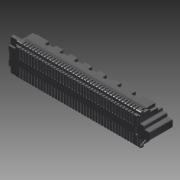
# Autodesk Inventor part: SS4-40_socket
Saved by Autodesk Inventor 2016 (Build 200138000, 138)
## iProperties
Category: PARTsolutions
Company: SAMTEC
Created: 2016-06-07
Part Number: SS4-40_socket
Catalog Web Link: www.cadenas.de
Description: SS4--Socket
Vendor: SAMTEC
Document SubType Name: Modeling
Designer: psAdmin
Manufacturer: SAMTEC
Mass: 0.109161 g
Surface Area: 7.02926 cm^2
Volume: 0.109161 cm^3
Density: 1 g/cm^3
Material: Generic
Appearance: PSOLRGB-175-175-175
PSOL_IDENT_0: {$CADENAS_DATA\23d-libs\samtec\modelling\ss4\parts\ss4_socket.prj},174 {VTYP=3D},{NB=SS4-40_socket},
PSOL_IDENT_1: {LINA=SS4-40_socket},{NN=SS4-},{DATE=07.12.2015 15:39:44},{GEOMDATE=07.12.2015 15:39:00},{VERSION=},
PSOL_IDENT_2: {LINEID=10},{LINESUBID=-1},{WBVAR=POS,LOPT}  {NB=SS4-40_socket},{LINA=SS4-40_socket},{KT=DUMMY},{PN=
PSOL_IDENT_3: SS4-40},{SERIES=SS4},{POSALG=   '10' , '-10' , '15' , '-15' , '20' , '-20' , '30' , '-30' , '40' , '
PSOL_IDENT_4: -40' ,  '50' , '-50'   },{POS=40},{ROPT=D},{LOPT=},{A=17.460},{BH=0.500},{K=2.725},{L=19.540},{W=4.3
PSOL_IDENT_5: 50},{HOLE=0.585},{PINS=40},{PINW=0.166},{PITCH=0.40},{LOPTPN=}
NN: SS4-
NT: Socket
NB: SS4-40_socket
NBSYN: $PN._socket
LINA: SS4-40_socket
PN: SS4-40
SERIES: SS4
POS: -40
ROPT: D
LOPT: Not Selected
A: 17.460
BH: 0.500
K: 2.725
L: 19.540
W: 4.350
HOLE: 0.585
PINW: 0.166
PITCH: 0.40
SUPPLIER: SAMTEC
ARTICLENO: SS4-40_socket
BOMINFO: SS4-40_socket
CREATOR: CADENAS GmbH
Title: SS4-40_socket
Author: Cadenas PARTsolutions
Comments: Socket
Autodesk Inventor part; units mm, degrees
sketch "Sketch_1" plane through (0, 0, 0) normal (0, 1, 0) x (1, 0, 0)
  line L0 (-9.56, -0.5) -> (-9.56, -2.175)
  line L1 (-9.56, -2.175) -> (8.58, -2.175)
  line L2 (8.58, -2.175) -> (8.58, -0.5)
  line L3 (8.58, -0.5) -> (8.18, -0.5)
  line L4 (8.18, -0.5) -> (8.18, 0.5)
  line L5 (8.18, 0.5) -> (8.58, 0.5)
  line L6 (8.58, 0.5) -> (8.58, 2.175)
  line L7 (8.58, 2.175) -> (-9.56, 2.175)
  line L8 (-9.56, 2.175) -> (-9.56, 0.5)
  line L9 (-9.56, 0.5) -> (-9.46, 0.5)
  line L10 (-9.46, 0.5) -> (-9.46, -0.5)
  line L11 (-9.46, -0.5) -> (-9.56, -0.5)
  line L12 (7.717, -0.705) -> (7.717, -1.29)
  line L13 (7.717, -1.29) -> (7.883, -1.29)
  line L14 (7.883, -1.29) -> (7.883, -0.705)
  line L15 (7.883, -0.705) -> (7.717, -0.705)
  line L16 (7.717, 1.29) -> (7.717, 0.705)
  line L17 (7.717, 0.705) -> (7.883, 0.705)
  line L18 (7.883, 0.705) -> (7.883, 1.29)
  line L19 (7.883, 1.29) -> (7.717, 1.29)
  line L20 (7.317, -0.705) -> (7.317, -1.29)
  line L21 (7.317, -1.29) -> (7.483, -1.29)
  line L22 (7.483, -1.29) -> (7.483, -0.705)
  line L23 (7.483, -0.705) -> (7.317, -0.705)
  line L24 (7.317, 1.29) -> (7.317, 0.705)
  line L25 (7.317, 0.705) -> (7.483, 0.705)
  line L26 (7.483, 0.705) -> (7.483, 1.29)
  line L27 (7.483, 1.29) -> (7.317, 1.29)
  line L28 (6.917, -0.705) -> (6.917, -1.29)
  line L29 (6.917, -1.29) -> (7.083, -1.29)
  line L30 (7.083, -1.29) -> (7.083, -0.705)
  line L31 (7.083, -0.705) -> (6.917, -0.705)
  line L32 (6.917, 1.29) -> (6.917, 0.705)
  line L33 (6.917, 0.705) -> (7.083, 0.705)
  line L34 (7.083, 0.705) -> (7.083, 1.29)
  line L35 (7.083, 1.29) -> (6.917, 1.29)
  line L36 (6.517, -0.705) -> (6.517, -1.29)
  line L37 (6.517, -1.29) -> (6.683, -1.29)
  line L38 (6.683, -1.29) -> (6.683, -0.705)
  line L39 (6.683, -0.705) -> (6.517, -0.705)
  line L40 (6.517, 1.29) -> (6.517, 0.705)
  line L41 (6.517, 0.705) -> (6.683, 0.705)
  line L42 (6.683, 0.705) -> (6.683, 1.29)
  line L43 (6.683, 1.29) -> (6.517, 1.29)
  line L44 (6.117, -0.705) -> (6.117, -1.29)
  line L45 (6.117, -1.29) -> (6.283, -1.29)
  line L46 (6.283, -1.29) -> (6.283, -0.705)
  line L47 (6.283, -0.705) -> (6.117, -0.705)
  line L48 (6.117, 1.29) -> (6.117, 0.705)
  line L49 (6.117, 0.705) -> (6.283, 0.705)
  line L50 (6.283, 0.705) -> (6.283, 1.29)
  line L51 (6.283, 1.29) -> (6.117, 1.29)
  line L52 (5.717, -0.705) -> (5.717, -1.29)
  line L53 (5.717, -1.29) -> (5.883, -1.29)
  line L54 (5.883, -1.29) -> (5.883, -0.705)
  line L55 (5.883, -0.705) -> (5.717, -0.705)
  line L56 (5.717, 1.29) -> (5.717, 0.705)
  line L57 (5.717, 0.705) -> (5.883, 0.705)
  line L58 (5.883, 0.705) -> (5.883, 1.29)
  line L59 (5.883, 1.29) -> (5.717, 1.29)
  line L60 (5.317, -0.705) -> (5.317, -1.29)
  line L61 (5.317, -1.29) -> (5.483, -1.29)
  line L62 (5.483, -1.29) -> (5.483, -0.705)
  line L63 (5.483, -0.705) -> (5.317, -0.705)
  line L64 (5.317, 1.29) -> (5.317, 0.705)
  line L65 (5.317, 0.705) -> (5.483, 0.705)
  line L66 (5.483, 0.705) -> (5.483, 1.29)
  line L67 (5.483, 1.29) -> (5.317, 1.29)
  line L68 (4.917, -0.705) -> (4.917, -1.29)
  line L69 (4.917, -1.29) -> (5.083, -1.29)
  line L70 (5.083, -1.29) -> (5.083, -0.705)
  line L71 (5.083, -0.705) -> (4.917, -0.705)
  line L72 (4.917, 1.29) -> (4.917, 0.705)
  line L73 (4.917, 0.705) -> (5.083, 0.705)
  line L74 (5.083, 0.705) -> (5.083, 1.29)
  line L75 (5.083, 1.29) -> (4.917, 1.29)
  line L76 (4.517, -0.705) -> (4.517, -1.29)
  line L77 (4.517, -1.29) -> (4.683, -1.29)
  line L78 (4.683, -1.29) -> (4.683, -0.705)
  line L79 (4.683, -0.705) -> (4.517, -0.705)
  line L80 (4.517, 1.29) -> (4.517, 0.705)
  line L81 (4.517, 0.705) -> (4.683, 0.705)
  line L82 (4.683, 0.705) -> (4.683, 1.29)
  line L83 (4.683, 1.29) -> (4.517, 1.29)
  line L84 (4.117, -0.705) -> (4.117, -1.29)
  line L85 (4.117, -1.29) -> (4.283, -1.29)
  line L86 (4.283, -1.29) -> (4.283, -0.705)
  line L87 (4.283, -0.705) -> (4.117, -0.705)
  line L88 (4.117, 1.29) -> (4.117, 0.705)
  line L89 (4.117, 0.705) -> (4.283, 0.705)
  line L90 (4.283, 0.705) -> (4.283, 1.29)
  line L91 (4.283, 1.29) -> (4.117, 1.29)
  line L92 (3.717, -0.705) -> (3.717, -1.29)
  line L93 (3.717, -1.29) -> (3.883, -1.29)
  line L94 (3.883, -1.29) -> (3.883, -0.705)
  line L95 (3.883, -0.705) -> (3.717, -0.705)
  line L96 (3.717, 1.29) -> (3.717, 0.705)
  line L97 (3.717, 0.705) -> (3.883, 0.705)
  line L98 (3.883, 0.705) -> (3.883, 1.29)
  line L99 (3.883, 1.29) -> (3.717, 1.29)
  line L100 (3.317, -0.705) -> (3.317, -1.29)
  line L101 (3.317, -1.29) -> (3.483, -1.29)
  line L102 (3.483, -1.29) -> (3.483, -0.705)
  line L103 (3.483, -0.705) -> (3.317, -0.705)
  line L104 (3.317, 1.29) -> (3.317, 0.705)
  line L105 (3.317, 0.705) -> (3.483, 0.705)
  line L106 (3.483, 0.705) -> (3.483, 1.29)
  line L107 (3.483, 1.29) -> (3.317, 1.29)
  line L108 (2.917, -0.705) -> (2.917, -1.29)
  line L109 (2.917, -1.29) -> (3.083, -1.29)
  line L110 (3.083, -1.29) -> (3.083, -0.705)
  line L111 (3.083, -0.705) -> (2.917, -0.705)
  line L112 (2.917, 1.29) -> (2.917, 0.705)
  line L113 (2.917, 0.705) -> (3.083, 0.705)
  line L114 (3.083, 0.705) -> (3.083, 1.29)
  line L115 (3.083, 1.29) -> (2.917, 1.29)
  line L116 (2.517, -0.705) -> (2.517, -1.29)
  line L117 (2.517, -1.29) -> (2.683, -1.29)
  line L118 (2.683, -1.29) -> (2.683, -0.705)
  line L119 (2.683, -0.705) -> (2.517, -0.705)
  line L120 (2.517, 1.29) -> (2.517, 0.705)
  line L121 (2.517, 0.705) -> (2.683, 0.705)
  line L122 (2.683, 0.705) -> (2.683, 1.29)
  line L123 (2.683, 1.29) -> (2.517, 1.29)
  line L124 (2.117, -0.705) -> (2.117, -1.29)
  line L125 (2.117, -1.29) -> (2.283, -1.29)
  line L126 (2.283, -1.29) -> (2.283, -0.705)
  line L127 (2.283, -0.705) -> (2.117, -0.705)
  line L128 (2.117, 1.29) -> (2.117, 0.705)
  line L129 (2.117, 0.705) -> (2.283, 0.705)
  line L130 (2.283, 0.705) -> (2.283, 1.29)
  line L131 (2.283, 1.29) -> (2.117, 1.29)
  line L132 (1.717, -0.705) -> (1.717, -1.29)
  line L133 (1.717, -1.29) -> (1.883, -1.29)
  line L134 (1.883, -1.29) -> (1.883, -0.705)
  line L135 (1.883, -0.705) -> (1.717, -0.705)
  line L136 (1.717, 1.29) -> (1.717, 0.705)
  line L137 (1.717, 0.705) -> (1.883, 0.705)
  line L138 (1.883, 0.705) -> (1.883, 1.29)
  line L139 (1.883, 1.29) -> (1.717, 1.29)
  line L140 (1.317, -0.705) -> (1.317, -1.29)
  line L141 (1.317, -1.29) -> (1.483, -1.29)
  line L142 (1.483, -1.29) -> (1.483, -0.705)
  line L143 (1.483, -0.705) -> (1.317, -0.705)
  line L144 (1.317, 1.29) -> (1.317, 0.705)
  line L145 (1.317, 0.705) -> (1.483, 0.705)
  line L146 (1.483, 0.705) -> (1.483, 1.29)
  line L147 (1.483, 1.29) -> (1.317, 1.29)
  line L148 (0.917, -0.705) -> (0.917, -1.29)
  line L149 (0.917, -1.29) -> (1.083, -1.29)
  line L150 (1.083, -1.29) -> (1.083, -0.705)
  line L151 (1.083, -0.705) -> (0.917, -0.705)
  line L152 (0.917, 1.29) -> (0.917, 0.705)
  line L153 (0.917, 0.705) -> (1.083, 0.705)
  line L154 (1.083, 0.705) -> (1.083, 1.29)
  line L155 (1.083, 1.29) -> (0.917, 1.29)
  line L156 (0.517, -0.705) -> (0.517, -1.29)
  line L157 (0.517, -1.29) -> (0.683, -1.29)
  line L158 (0.683, -1.29) -> (0.683, -0.705)
  line L159 (0.683, -0.705) -> (0.517, -0.705)
  line L160 (0.517, 1.29) -> (0.517, 0.705)
  line L161 (0.517, 0.705) -> (0.683, 0.705)
  line L162 (0.683, 0.705) -> (0.683, 1.29)
  line L163 (0.683, 1.29) -> (0.517, 1.29)
  line L164 (0.117, -0.705) -> (0.117, -1.29)
  line L165 (0.117, -1.29) -> (0.283, -1.29)
  line L166 (0.283, -1.29) -> (0.283, -0.705)
  line L167 (0.283, -0.705) -> (0.117, -0.705)
  line L168 (0.117, 1.29) -> (0.117, 0.705)
  line L169 (0.117, 0.705) -> (0.283, 0.705)
  line L170 (0.283, 0.705) -> (0.283, 1.29)
  line L171 (0.283, 1.29) -> (0.117, 1.29)
  line L172 (-0.283, -0.705) -> (-0.283, -1.29)
  line L173 (-0.283, -1.29) -> (-0.117, -1.29)
  line L174 (-0.117, -1.29) -> (-0.117, -0.705)
  line L175 (-0.117, -0.705) -> (-0.283, -0.705)
  line L176 (-0.283, 1.29) -> (-0.283, 0.705)
  line L177 (-0.283, 0.705) -> (-0.117, 0.705)
  line L178 (-0.117, 0.705) -> (-0.117, 1.29)
  line L179 (-0.117, 1.29) -> (-0.283, 1.29)
  line L180 (-0.683, -0.705) -> (-0.683, -1.29)
  line L181 (-0.683, -1.29) -> (-0.517, -1.29)
  line L182 (-0.517, -1.29) -> (-0.517, -0.705)
  line L183 (-0.517, -0.705) -> (-0.683, -0.705)
  line L184 (-0.683, 1.29) -> (-0.683, 0.705)
  line L185 (-0.683, 0.705) -> (-0.517, 0.705)
  line L186 (-0.517, 0.705) -> (-0.517, 1.29)
  line L187 (-0.517, 1.29) -> (-0.683, 1.29)
  line L188 (-1.083, -0.705) -> (-1.083, -1.29)
  line L189 (-1.083, -1.29) -> (-0.917, -1.29)
  line L190 (-0.917, -1.29) -> (-0.917, -0.705)
  line L191 (-0.917, -0.705) -> (-1.083, -0.705)
  line L192 (-1.083, 1.29) -> (-1.083, 0.705)
  line L193 (-1.083, 0.705) -> (-0.917, 0.705)
  line L194 (-0.917, 0.705) -> (-0.917, 1.29)
  line L195 (-0.917, 1.29) -> (-1.083, 1.29)
  line L196 (-1.483, -0.705) -> (-1.483, -1.29)
  line L197 (-1.483, -1.29) -> (-1.317, -1.29)
  line L198 (-1.317, -1.29) -> (-1.317, -0.705)
  line L199 (-1.317, -0.705) -> (-1.483, -0.705)
  line L200 (-1.483, 1.29) -> (-1.483, 0.705)
  line L201 (-1.483, 0.705) -> (-1.317, 0.705)
  line L202 (-1.317, 0.705) -> (-1.317, 1.29)
  line L203 (-1.317, 1.29) -> (-1.483, 1.29)
  line L204 (-1.883, -0.705) -> (-1.883, -1.29)
  line L205 (-1.883, -1.29) -> (-1.717, -1.29)
  line L206 (-1.717, -1.29) -> (-1.717, -0.705)
  line L207 (-1.717, -0.705) -> (-1.883, -0.705)
  line L208 (-1.883, 1.29) -> (-1.883, 0.705)
  line L209 (-1.883, 0.705) -> (-1.717, 0.705)
  line L210 (-1.717, 0.705) -> (-1.717, 1.29)
  line L211 (-1.717, 1.29) -> (-1.883, 1.29)
  line L212 (-2.283, -0.705) -> (-2.283, -1.29)
  line L213 (-2.283, -1.29) -> (-2.117, -1.29)
  line L214 (-2.117, -1.29) -> (-2.117, -0.705)
  line L215 (-2.117, -0.705) -> (-2.283, -0.705)
  line L216 (-2.283, 1.29) -> (-2.283, 0.705)
  line L217 (-2.283, 0.705) -> (-2.117, 0.705)
  line L218 (-2.117, 0.705) -> (-2.117, 1.29)
  line L219 (-2.117, 1.29) -> (-2.283, 1.29)
  line L220 (-2.683, -0.705) -> (-2.683, -1.29)
  line L221 (-2.683, -1.29) -> (-2.517, -1.29)
  line L222 (-2.517, -1.29) -> (-2.517, -0.705)
  line L223 (-2.517, -0.705) -> (-2.683, -0.705)
  line L224 (-2.683, 1.29) -> (-2.683, 0.705)
  line L225 (-2.683, 0.705) -> (-2.517, 0.705)
  line L226 (-2.517, 0.705) -> (-2.517, 1.29)
  line L227 (-2.517, 1.29) -> (-2.683, 1.29)
  line L228 (-3.083, -0.705) -> (-3.083, -1.29)
  line L229 (-3.083, -1.29) -> (-2.917, -1.29)
  line L230 (-2.917, -1.29) -> (-2.917, -0.705)
  line L231 (-2.917, -0.705) -> (-3.083, -0.705)
  line L232 (-3.083, 1.29) -> (-3.083, 0.705)
  line L233 (-3.083, 0.705) -> (-2.917, 0.705)
  line L234 (-2.917, 0.705) -> (-2.917, 1.29)
  line L235 (-2.917, 1.29) -> (-3.083, 1.29)
  line L236 (-3.483, -0.705) -> (-3.483, -1.29)
  line L237 (-3.483, -1.29) -> (-3.317, -1.29)
  line L238 (-3.317, -1.29) -> (-3.317, -0.705)
  line L239 (-3.317, -0.705) -> (-3.483, -0.705)
  line L240 (-3.483, 1.29) -> (-3.483, 0.705)
  line L241 (-3.483, 0.705) -> (-3.317, 0.705)
  line L242 (-3.317, 0.705) -> (-3.317, 1.29)
  line L243 (-3.317, 1.29) -> (-3.483, 1.29)
  line L244 (-3.883, -0.705) -> (-3.883, -1.29)
  line L245 (-3.883, -1.29) -> (-3.717, -1.29)
  line L246 (-3.717, -1.29) -> (-3.717, -0.705)
  line L247 (-3.717, -0.705) -> (-3.883, -0.705)
  line L248 (-3.883, 1.29) -> (-3.883, 0.705)
  line L249 (-3.883, 0.705) -> (-3.717, 0.705)
  line L250 (-3.717, 0.705) -> (-3.717, 1.29)
  line L251 (-3.717, 1.29) -> (-3.883, 1.29)
  line L252 (-4.283, -0.705) -> (-4.283, -1.29)
  line L253 (-4.283, -1.29) -> (-4.117, -1.29)
  line L254 (-4.117, -1.29) -> (-4.117, -0.705)
  line L255 (-4.117, -0.705) -> (-4.283, -0.705)
  line L256 (-4.283, 1.29) -> (-4.283, 0.705)
  line L257 (-4.283, 0.705) -> (-4.117, 0.705)
  line L258 (-4.117, 0.705) -> (-4.117, 1.29)
  line L259 (-4.117, 1.29) -> (-4.283, 1.29)
  line L260 (-4.683, -0.705) -> (-4.683, -1.29)
  line L261 (-4.683, -1.29) -> (-4.517, -1.29)
  line L262 (-4.517, -1.29) -> (-4.517, -0.705)
  line L263 (-4.517, -0.705) -> (-4.683, -0.705)
  line L264 (-4.683, 1.29) -> (-4.683, 0.705)
  line L265 (-4.683, 0.705) -> (-4.517, 0.705)
  line L266 (-4.517, 0.705) -> (-4.517, 1.29)
  line L267 (-4.517, 1.29) -> (-4.683, 1.29)
  line L268 (-5.083, -0.705) -> (-5.083, -1.29)
  line L269 (-5.083, -1.29) -> (-4.917, -1.29)
  line L270 (-4.917, -1.29) -> (-4.917, -0.705)
  line L271 (-4.917, -0.705) -> (-5.083, -0.705)
  line L272 (-5.083, 1.29) -> (-5.083, 0.705)
  line L273 (-5.083, 0.705) -> (-4.917, 0.705)
  line L274 (-4.917, 0.705) -> (-4.917, 1.29)
  line L275 (-4.917, 1.29) -> (-5.083, 1.29)
  line L276 (-5.483, -0.705) -> (-5.483, -1.29)
  line L277 (-5.483, -1.29) -> (-5.317, -1.29)
  line L278 (-5.317, -1.29) -> (-5.317, -0.705)
  line L279 (-5.317, -0.705) -> (-5.483, -0.705)
  line L280 (-5.483, 1.29) -> (-5.483, 0.705)
  line L281 (-5.483, 0.705) -> (-5.317, 0.705)
  line L282 (-5.317, 0.705) -> (-5.317, 1.29)
  line L283 (-5.317, 1.29) -> (-5.483, 1.29)
  line L284 (-5.883, -0.705) -> (-5.883, -1.29)
  line L285 (-5.883, -1.29) -> (-5.717, -1.29)
  line L286 (-5.717, -1.29) -> (-5.717, -0.705)
  line L287 (-5.717, -0.705) -> (-5.883, -0.705)
  line L288 (-5.883, 1.29) -> (-5.883, 0.705)
  line L289 (-5.883, 0.705) -> (-5.717, 0.705)
  line L290 (-5.717, 0.705) -> (-5.717, 1.29)
  line L291 (-5.717, 1.29) -> (-5.883, 1.29)
  line L292 (-6.283, -0.705) -> (-6.283, -1.29)
  line L293 (-6.283, -1.29) -> (-6.117, -1.29)
  line L294 (-6.117, -1.29) -> (-6.117, -0.705)
  line L295 (-6.117, -0.705) -> (-6.283, -0.705)
  line L296 (-6.283, 1.29) -> (-6.283, 0.705)
  line L297 (-6.283, 0.705) -> (-6.117, 0.705)
  line L298 (-6.117, 0.705) -> (-6.117, 1.29)
  line L299 (-6.117, 1.29) -> (-6.283, 1.29)
  line L300 (-6.683, -0.705) -> (-6.683, -1.29)
  line L301 (-6.683, -1.29) -> (-6.517, -1.29)
  line L302 (-6.517, -1.29) -> (-6.517, -0.705)
  line L303 (-6.517, -0.705) -> (-6.683, -0.705)
  line L304 (-6.683, 1.29) -> (-6.683, 0.705)
  line L305 (-6.683, 0.705) -> (-6.517, 0.705)
  line L306 (-6.517, 0.705) -> (-6.517, 1.29)
  line L307 (-6.517, 1.29) -> (-6.683, 1.29)
  line L308 (-7.083, -0.705) -> (-7.083, -1.29)
  line L309 (-7.083, -1.29) -> (-6.917, -1.29)
  line L310 (-6.917, -1.29) -> (-6.917, -0.705)
  line L311 (-6.917, -0.705) -> (-7.083, -0.705)
  line L312 (-7.083, 1.29) -> (-7.083, 0.705)
  line L313 (-7.083, 0.705) -> (-6.917, 0.705)
  line L314 (-6.917, 0.705) -> (-6.917, 1.29)
  line L315 (-6.917, 1.29) -> (-7.083, 1.29)
  line L316 (-7.483, -0.705) -> (-7.483, -1.29)
  line L317 (-7.483, -1.29) -> (-7.317, -1.29)
  line L318 (-7.317, -1.29) -> (-7.317, -0.705)
  line L319 (-7.317, -0.705) -> (-7.483, -0.705)
  line L320 (-7.483, 1.29) -> (-7.483, 0.705)
  line L321 (-7.483, 0.705) -> (-7.317, 0.705)
  line L322 (-7.317, 0.705) -> (-7.317, 1.29)
  line L323 (-7.317, 1.29) -> (-7.483, 1.29)
  line L324 (-7.883, -0.705) -> (-7.883, -1.29)
  line L325 (-7.883, -1.29) -> (-7.717, -1.29)
  line L326 (-7.717, -1.29) -> (-7.717, -0.705)
  line L327 (-7.717, -0.705) -> (-7.883, -0.705)
  line L328 (-7.883, 1.29) -> (-7.883, 0.705)
  line L329 (-7.883, 0.705) -> (-7.717, 0.705)
  line L330 (-7.717, 0.705) -> (-7.717, 1.29)
  line L331 (-7.717, 1.29) -> (-7.883, 1.29)
  constraints: 664 end point
extrude "Extrusion1" add sketch "Sketch_1" along normal blind 2.725
sketch "Sketch_5" plane through (0, 0, 0) normal (0, 0, 1) x (1, 0, 0)
  line L0 (-9.56, 0.2) -> (-9.56, -0.4)
  line L1 (-9.56, -0.4) -> (8.58, -0.4)
  line L2 (8.58, -0.4) -> (8.58, 0.2)
  line L3 (8.58, 0.2) -> (8.38, 0.2)
  line L4 (8.38, 0.2) -> (8.38, 0)
  line L5 (8.38, 0) -> (-8.36, 0)
  line L6 (-8.36, 0) -> (-8.36, 0.2)
  line L7 (-8.36, 0.2) -> (-9.56, 0.2)
  constraints: 16 end point
extrude "Extrusion2" cut sketch "Sketch_5" along normal mid plane 4.35
sketch "Sketch_6" plane through (0, 0.9, 0) normal (0, 1, 0) x (1, 0, 0)
  line L0 (-9.56, 2.175) -> (-9.56, -2.175)
  line L1 (-9.56, -2.175) -> (-8.56, -2.175)
  line L2 (-8.56, -2.175) -> (-8.56, 2.175)
  line L3 (-8.56, 2.175) -> (-9.56, 2.175)
  constraints: 8 end point
extrude "Extrusion3" cut sketch "Sketch_6" along normal blind 3
sketch "Sketch_7" plane through (0, 0.9, 0) normal (0, 1, 0) x (1, 0, 0)
  line L0 (-9.56, -0.5) -> (-9.56, -0.955)
  arc A0 (-9.56, -0.955) -> (-9.31, -1.205) centre (-9.31, -0.955) ccw
  line L1 (-9.31, -1.205) -> (-8.16, -1.205)
  line L2 (-8.16, -1.205) -> (-8.16, 1.205)
  line L3 (-8.16, 1.205) -> (-9.31, 1.205)
  arc A1 (-9.31, 1.205) -> (-9.56, 0.955) centre (-9.31, 0.955) ccw
  line L4 (-9.56, 0.955) -> (-9.56, 0.5)
  line L5 (-9.56, 0.5) -> (-9.46, 0.5)
  line L6 (-9.46, 0.5) -> (-9.46, -0.5)
  line L7 (-9.46, -0.5) -> (-9.56, -0.5)
  constraints: 16 end point, 4 point on circle, 2 centre point
extrude "Extrusion4" add sketch "Sketch_7" along normal blind 2.48
sketch "Sketch_9" plane through (0, 0.2, 0) normal (0, 1, 0) x (1, 0, 0)
  line L0 (8.18, -1.2) -> (8.58, -1.2)
  line L1 (8.58, -1.2) -> (8.58, -0.9)
  line L2 (8.58, -0.9) -> (9.08, -0.9)
  arc A0 (9.08, -0.9) -> (9.23, -0.75) centre (9.08, -0.75) ccw
  line L3 (9.23, -0.75) -> (9.23, -0.6)
  arc A1 (9.33, -0.5) -> (9.23, -0.6) centre (9.33, -0.6) ccw
  line L4 (9.33, -0.5) -> (9.83, -0.5)
  arc A2 (9.83, -0.5) -> (9.98, -0.35) centre (9.83, -0.35) ccw
  line L5 (9.98, -0.35) -> (9.98, 0.346)
  arc A3 (9.98, 0.346) -> (9.826, 0.5) centre (9.826, 0.346) ccw
  line L6 (9.826, 0.5) -> (9.33, 0.5)
  arc A4 (9.23, 0.6) -> (9.33, 0.5) centre (9.33, 0.6) ccw
  line L7 (9.23, 0.6) -> (9.23, 0.75)
  arc A5 (9.23, 0.75) -> (9.08, 0.9) centre (9.08, 0.75) ccw
  line L8 (9.08, 0.9) -> (8.58, 0.9)
  line L9 (8.58, 0.9) -> (8.58, 1.2)
  line L10 (8.58, 1.2) -> (8.18, 1.2)
  line L11 (8.18, 1.2) -> (8.18, -1.2)
  constraints: 24 end point, 12 point on circle, 6 centre point
extrude "Extrusion5" add sketch "Sketch_9" along normal blind 0.4
sketch "Sketch_11" plane through (-8.16, 0, 0) normal (1, 0, 0) x (0, 0, -1)
  line L0 (-1.025, 2.725) -> (-0.775, 2.368)
  line L1 (-0.775, 2.368) -> (-0.775, 0.9431)
  line L2 (-0.775, 0.9431) -> (-0.705, 0.6818)
  arc A0 (-0.705, 0.6818) -> (-0.52, 0.6) centre (-0.52, 0.85) ccw
  line L3 (-0.52, 0.6) -> (0.52, 0.6)
  arc A1 (0.52, 0.6) -> (0.705, 0.6818) centre (0.52, 0.85) ccw
  line L4 (0.705, 0.6818) -> (0.775, 0.9431)
  line L5 (0.775, 0.9431) -> (0.775, 2.368)
  line L6 (0.775, 2.368) -> (1.025, 2.725)
  line L7 (1.025, 2.725) -> (-1.025, 2.725)
  constraints: 16 end point, 4 point on circle, 2 centre point
extrude "Extrusion6" cut sketch "Sketch_11" along normal blind 16.34
sketch "Sketch_12" plane through (0, 0.2, 0) normal (0, 1, 0) x (1, 0, 0)
  line L0 (8.18, 0.5) -> (8.73, 0.5)
  line L1 (8.73, 0.5) -> (8.73, -0.5)
  line L2 (8.73, -0.5) -> (8.18, -0.5)
  line L3 (8.18, -0.5) -> (8.18, -1.205)
  line L4 (8.18, -1.205) -> (8.58, -1.205)
  line L5 (8.58, -1.205) -> (8.58, -1.05)
  arc A0 (8.73, -0.9) -> (8.58, -1.05) centre (8.73, -1.05) ccw
  line L6 (8.73, -0.9) -> (9.08, -0.9)
  arc A1 (9.08, -0.9) -> (9.23, -0.75) centre (9.08, -0.75) ccw
  line L7 (9.23, -0.75) -> (9.23, -0.6)
  arc A2 (9.33, -0.5) -> (9.23, -0.6) centre (9.33, -0.6) ccw
  line L8 (9.33, -0.5) -> (9.83, -0.5)
  arc A3 (9.83, -0.5) -> (9.98, -0.35) centre (9.83, -0.35) ccw
  line L9 (9.98, -0.35) -> (9.98, 0.346)
  arc A4 (9.98, 0.346) -> (9.826, 0.5) centre (9.826, 0.346) ccw
  line L10 (9.826, 0.5) -> (9.33, 0.5)
  arc A5 (9.23, 0.6) -> (9.33, 0.5) centre (9.33, 0.6) ccw
  line L11 (9.23, 0.6) -> (9.23, 0.75)
  arc A6 (9.23, 0.75) -> (9.08, 0.9) centre (9.08, 0.75) ccw
  line L12 (9.08, 0.9) -> (8.73, 0.9)
  arc A7 (8.58, 1.05) -> (8.73, 0.9) centre (8.73, 1.05) ccw
  line L13 (8.58, 1.05) -> (8.58, 1.205)
  line L14 (8.58, 1.205) -> (8.18, 1.205)
  line L15 (8.18, 1.205) -> (8.18, 0.5)
  constraints: 32 end point, 16 point on circle, 8 centre point
extrude "Extrusion7" add sketch "Sketch_12" along normal blind 3.18
sketch "Sketch_14" plane through (0, 0, 0) normal (1, 0, 0) x (0, 0, -1)
  line L0 (-0.877, 3.38) -> (-0.707, 3.0856)
  line L1 (-0.707, 3.0856) -> (-0.707, 1.0801)
  line L2 (-0.707, 1.0801) -> (-0.6319, 0.8)
  arc A0 (-0.6319, 0.8) -> (-0.387, 0.6) centre (-0.387, 0.85) ccw
  line L3 (-0.387, 0.6) -> (0.387, 0.6)
  arc A1 (0.387, 0.6) -> (0.6319, 0.8) centre (0.387, 0.85) ccw
  line L4 (0.6319, 0.8) -> (0.707, 1.0801)
  line L5 (0.707, 1.0801) -> (0.707, 3.0856)
  line L6 (0.707, 3.0856) -> (0.877, 3.38)
  line L7 (0.877, 3.38) -> (-0.877, 3.38)
  constraints: 16 end point, 4 point on circle, 2 centre point
extrude "Extrusion8" cut sketch "Sketch_14" against normal blind 8.73
sketch "Sketch_16" plane through (0, 0, 0) normal (0, 0, 1) x (1, 0, 0)
  line L0 (-8.33, 3.38) -> (-8.16, 3.0856)
  line L1 (-8.16, 3.0856) -> (-8.16, 2.725)
  line L2 (-8.16, 2.725) -> (8.18, 2.725)
  line L3 (8.18, 2.725) -> (8.18, 3.0856)
  line L4 (8.18, 3.0856) -> (8.35, 3.38)
  line L5 (8.35, 3.38) -> (-8.33, 3.38)
  constraints: 12 end point
extrude "Extrusion9" cut sketch "Sketch_16" along normal mid plane 4.35
sketch "Sketch_18" plane through (0, 0, 2.175) normal (0, 0, 1) x (1, 0, 0)
  line L0 (-7.883, -1) -> (8.117, -1)
  line L1 (8.117, -1) -> (8.117, -0.25)
  line L2 (8.117, -0.25) -> (7.883, -0.25)
  line L3 (7.883, -0.25) -> (7.883, 0.95)
  line L4 (7.883, 0.95) -> (7.717, 0.95)
  line L5 (7.717, 0.95) -> (7.717, -0.25)
  line L6 (7.717, -0.25) -> (7.483, -0.25)
  line L7 (7.483, -0.25) -> (7.483, 0.95)
  line L8 (7.483, 0.95) -> (7.317, 0.95)
  line L9 (7.317, 0.95) -> (7.317, -0.25)
  line L10 (7.317, -0.25) -> (7.083, -0.25)
  line L11 (7.083, -0.25) -> (7.083, 0.95)
  line L12 (7.083, 0.95) -> (6.917, 0.95)
  line L13 (6.917, 0.95) -> (6.917, -0.25)
  line L14 (6.917, -0.25) -> (6.683, -0.25)
  line L15 (6.683, -0.25) -> (6.683, 0.95)
  line L16 (6.683, 0.95) -> (6.517, 0.95)
  line L17 (6.517, 0.95) -> (6.517, -0.25)
  line L18 (6.517, -0.25) -> (6.283, -0.25)
  line L19 (6.283, -0.25) -> (6.283, 0.95)
  line L20 (6.283, 0.95) -> (6.117, 0.95)
  line L21 (6.117, 0.95) -> (6.117, -0.25)
  line L22 (6.117, -0.25) -> (5.883, -0.25)
  line L23 (5.883, -0.25) -> (5.883, 0.95)
  line L24 (5.883, 0.95) -> (5.717, 0.95)
  line L25 (5.717, 0.95) -> (5.717, -0.25)
  line L26 (5.717, -0.25) -> (5.483, -0.25)
  line L27 (5.483, -0.25) -> (5.483, 0.95)
  line L28 (5.483, 0.95) -> (5.317, 0.95)
  line L29 (5.317, 0.95) -> (5.317, -0.25)
  line L30 (5.317, -0.25) -> (5.083, -0.25)
  line L31 (5.083, -0.25) -> (5.083, 0.95)
  line L32 (5.083, 0.95) -> (4.917, 0.95)
  line L33 (4.917, 0.95) -> (4.917, -0.25)
  line L34 (4.917, -0.25) -> (4.683, -0.25)
  line L35 (4.683, -0.25) -> (4.683, 0.95)
  line L36 (4.683, 0.95) -> (4.517, 0.95)
  line L37 (4.517, 0.95) -> (4.517, -0.25)
  line L38 (4.517, -0.25) -> (4.283, -0.25)
  line L39 (4.283, -0.25) -> (4.283, 0.95)
  line L40 (4.283, 0.95) -> (4.117, 0.95)
  line L41 (4.117, 0.95) -> (4.117, -0.25)
  line L42 (4.117, -0.25) -> (3.883, -0.25)
  line L43 (3.883, -0.25) -> (3.883, 0.95)
  line L44 (3.883, 0.95) -> (3.717, 0.95)
  line L45 (3.717, 0.95) -> (3.717, -0.25)
  line L46 (3.717, -0.25) -> (3.483, -0.25)
  line L47 (3.483, -0.25) -> (3.483, 0.95)
  line L48 (3.483, 0.95) -> (3.317, 0.95)
  line L49 (3.317, 0.95) -> (3.317, -0.25)
  line L50 (3.317, -0.25) -> (3.083, -0.25)
  line L51 (3.083, -0.25) -> (3.083, 0.95)
  line L52 (3.083, 0.95) -> (2.917, 0.95)
  line L53 (2.917, 0.95) -> (2.917, -0.25)
  line L54 (2.917, -0.25) -> (2.683, -0.25)
  line L55 (2.683, -0.25) -> (2.683, 0.95)
  line L56 (2.683, 0.95) -> (2.517, 0.95)
  line L57 (2.517, 0.95) -> (2.517, -0.25)
  line L58 (2.517, -0.25) -> (2.283, -0.25)
  line L59 (2.283, -0.25) -> (2.283, 0.95)
  line L60 (2.283, 0.95) -> (2.117, 0.95)
  line L61 (2.117, 0.95) -> (2.117, -0.25)
  line L62 (2.117, -0.25) -> (1.883, -0.25)
  line L63 (1.883, -0.25) -> (1.883, 0.95)
  line L64 (1.883, 0.95) -> (1.717, 0.95)
  line L65 (1.717, 0.95) -> (1.717, -0.25)
  line L66 (1.717, -0.25) -> (1.483, -0.25)
  line L67 (1.483, -0.25) -> (1.483, 0.95)
  line L68 (1.483, 0.95) -> (1.317, 0.95)
  line L69 (1.317, 0.95) -> (1.317, -0.25)
  line L70 (1.317, -0.25) -> (1.083, -0.25)
  line L71 (1.083, -0.25) -> (1.083, 0.95)
  line L72 (1.083, 0.95) -> (0.917, 0.95)
  line L73 (0.917, 0.95) -> (0.917, -0.25)
  line L74 (0.917, -0.25) -> (0.683, -0.25)
  line L75 (0.683, -0.25) -> (0.683, 0.95)
  line L76 (0.683, 0.95) -> (0.517, 0.95)
  line L77 (0.517, 0.95) -> (0.517, -0.25)
  line L78 (0.517, -0.25) -> (0.283, -0.25)
  line L79 (0.283, -0.25) -> (0.283, 0.95)
  line L80 (0.283, 0.95) -> (0.117, 0.95)
  line L81 (0.117, 0.95) -> (0.117, -0.25)
  line L82 (0.117, -0.25) -> (-0.117, -0.25)
  line L83 (-0.117, -0.25) -> (-0.117, 0.95)
  line L84 (-0.117, 0.95) -> (-0.283, 0.95)
  line L85 (-0.283, 0.95) -> (-0.283, -0.25)
  line L86 (-0.283, -0.25) -> (-0.517, -0.25)
  line L87 (-0.517, -0.25) -> (-0.517, 0.95)
  line L88 (-0.517, 0.95) -> (-0.683, 0.95)
  line L89 (-0.683, 0.95) -> (-0.683, -0.25)
  line L90 (-0.683, -0.25) -> (-0.917, -0.25)
  line L91 (-0.917, -0.25) -> (-0.917, 0.95)
  line L92 (-0.917, 0.95) -> (-1.083, 0.95)
  line L93 (-1.083, 0.95) -> (-1.083, -0.25)
  line L94 (-1.083, -0.25) -> (-1.317, -0.25)
  line L95 (-1.317, -0.25) -> (-1.317, 0.95)
  line L96 (-1.317, 0.95) -> (-1.483, 0.95)
  line L97 (-1.483, 0.95) -> (-1.483, -0.25)
  line L98 (-1.483, -0.25) -> (-1.717, -0.25)
  line L99 (-1.717, -0.25) -> (-1.717, 0.95)
  line L100 (-1.717, 0.95) -> (-1.883, 0.95)
  line L101 (-1.883, 0.95) -> (-1.883, -0.25)
  line L102 (-1.883, -0.25) -> (-2.117, -0.25)
  line L103 (-2.117, -0.25) -> (-2.117, 0.95)
  line L104 (-2.117, 0.95) -> (-2.283, 0.95)
  line L105 (-2.283, 0.95) -> (-2.283, -0.25)
  line L106 (-2.283, -0.25) -> (-2.517, -0.25)
  line L107 (-2.517, -0.25) -> (-2.517, 0.95)
  line L108 (-2.517, 0.95) -> (-2.683, 0.95)
  line L109 (-2.683, 0.95) -> (-2.683, -0.25)
  line L110 (-2.683, -0.25) -> (-2.917, -0.25)
  line L111 (-2.917, -0.25) -> (-2.917, 0.95)
  line L112 (-2.917, 0.95) -> (-3.083, 0.95)
  line L113 (-3.083, 0.95) -> (-3.083, -0.25)
  line L114 (-3.083, -0.25) -> (-3.317, -0.25)
  line L115 (-3.317, -0.25) -> (-3.317, 0.95)
  line L116 (-3.317, 0.95) -> (-3.483, 0.95)
  line L117 (-3.483, 0.95) -> (-3.483, -0.25)
  line L118 (-3.483, -0.25) -> (-3.717, -0.25)
  line L119 (-3.717, -0.25) -> (-3.717, 0.95)
  line L120 (-3.717, 0.95) -> (-3.883, 0.95)
  line L121 (-3.883, 0.95) -> (-3.883, -0.25)
  line L122 (-3.883, -0.25) -> (-4.117, -0.25)
  line L123 (-4.117, -0.25) -> (-4.117, 0.95)
  line L124 (-4.117, 0.95) -> (-4.283, 0.95)
  line L125 (-4.283, 0.95) -> (-4.283, -0.25)
  line L126 (-4.283, -0.25) -> (-4.517, -0.25)
  line L127 (-4.517, -0.25) -> (-4.517, 0.95)
  line L128 (-4.517, 0.95) -> (-4.683, 0.95)
  line L129 (-4.683, 0.95) -> (-4.683, -0.25)
  line L130 (-4.683, -0.25) -> (-4.917, -0.25)
  line L131 (-4.917, -0.25) -> (-4.917, 0.95)
  line L132 (-4.917, 0.95) -> (-5.083, 0.95)
  line L133 (-5.083, 0.95) -> (-5.083, -0.25)
  line L134 (-5.083, -0.25) -> (-5.317, -0.25)
  line L135 (-5.317, -0.25) -> (-5.317, 0.95)
  line L136 (-5.317, 0.95) -> (-5.483, 0.95)
  line L137 (-5.483, 0.95) -> (-5.483, -0.25)
  line L138 (-5.483, -0.25) -> (-5.717, -0.25)
  line L139 (-5.717, -0.25) -> (-5.717, 0.95)
  line L140 (-5.717, 0.95) -> (-5.883, 0.95)
  line L141 (-5.883, 0.95) -> (-5.883, -0.25)
  line L142 (-5.883, -0.25) -> (-6.117, -0.25)
  line L143 (-6.117, -0.25) -> (-6.117, 0.95)
  line L144 (-6.117, 0.95) -> (-6.283, 0.95)
  line L145 (-6.283, 0.95) -> (-6.283, -0.25)
  line L146 (-6.283, -0.25) -> (-6.517, -0.25)
  line L147 (-6.517, -0.25) -> (-6.517, 0.95)
  line L148 (-6.517, 0.95) -> (-6.683, 0.95)
  line L149 (-6.683, 0.95) -> (-6.683, -0.25)
  line L150 (-6.683, -0.25) -> (-6.917, -0.25)
  line L151 (-6.917, -0.25) -> (-6.917, 0.95)
  line L152 (-6.917, 0.95) -> (-7.083, 0.95)
  line L153 (-7.083, 0.95) -> (-7.083, -0.25)
  line L154 (-7.083, -0.25) -> (-7.317, -0.25)
  line L155 (-7.317, -0.25) -> (-7.317, 0.95)
  line L156 (-7.317, 0.95) -> (-7.483, 0.95)
  line L157 (-7.483, 0.95) -> (-7.483, -0.25)
  line L158 (-7.483, -0.25) -> (-7.717, -0.25)
  line L159 (-7.717, -0.25) -> (-7.717, 0.95)
  line L160 (-7.717, 0.95) -> (-7.883, 0.95)
  line L161 (-7.883, 0.95) -> (-7.883, -1)
  constraints: 324 end point
extrude "Extrusion10" cut sketch "Sketch_18" against normal blind 1.7
sketch "Sketch_19" plane through (0, 0, -2.175) normal (0, 0, 1) x (1, 0, 0)
  line L0 (-7.883, -1) -> (8.117, -1)
  line L1 (8.117, -1) -> (8.117, -0.25)
  line L2 (8.117, -0.25) -> (7.883, -0.25)
  line L3 (7.883, -0.25) -> (7.883, 0.95)
  line L4 (7.883, 0.95) -> (7.717, 0.95)
  line L5 (7.717, 0.95) -> (7.717, -0.25)
  line L6 (7.717, -0.25) -> (7.483, -0.25)
  line L7 (7.483, -0.25) -> (7.483, 0.95)
  line L8 (7.483, 0.95) -> (7.317, 0.95)
  line L9 (7.317, 0.95) -> (7.317, -0.25)
  line L10 (7.317, -0.25) -> (7.083, -0.25)
  line L11 (7.083, -0.25) -> (7.083, 0.95)
  line L12 (7.083, 0.95) -> (6.917, 0.95)
  line L13 (6.917, 0.95) -> (6.917, -0.25)
  line L14 (6.917, -0.25) -> (6.683, -0.25)
  line L15 (6.683, -0.25) -> (6.683, 0.95)
  line L16 (6.683, 0.95) -> (6.517, 0.95)
  line L17 (6.517, 0.95) -> (6.517, -0.25)
  line L18 (6.517, -0.25) -> (6.283, -0.25)
  line L19 (6.283, -0.25) -> (6.283, 0.95)
  line L20 (6.283, 0.95) -> (6.117, 0.95)
  line L21 (6.117, 0.95) -> (6.117, -0.25)
  line L22 (6.117, -0.25) -> (5.883, -0.25)
  line L23 (5.883, -0.25) -> (5.883, 0.95)
  line L24 (5.883, 0.95) -> (5.717, 0.95)
  line L25 (5.717, 0.95) -> (5.717, -0.25)
  line L26 (5.717, -0.25) -> (5.483, -0.25)
  line L27 (5.483, -0.25) -> (5.483, 0.95)
  line L28 (5.483, 0.95) -> (5.317, 0.95)
  line L29 (5.317, 0.95) -> (5.317, -0.25)
  line L30 (5.317, -0.25) -> (5.083, -0.25)
  line L31 (5.083, -0.25) -> (5.083, 0.95)
  line L32 (5.083, 0.95) -> (4.917, 0.95)
  line L33 (4.917, 0.95) -> (4.917, -0.25)
  line L34 (4.917, -0.25) -> (4.683, -0.25)
  line L35 (4.683, -0.25) -> (4.683, 0.95)
  line L36 (4.683, 0.95) -> (4.517, 0.95)
  line L37 (4.517, 0.95) -> (4.517, -0.25)
  line L38 (4.517, -0.25) -> (4.283, -0.25)
  line L39 (4.283, -0.25) -> (4.283, 0.95)
  line L40 (4.283, 0.95) -> (4.117, 0.95)
  line L41 (4.117, 0.95) -> (4.117, -0.25)
  line L42 (4.117, -0.25) -> (3.883, -0.25)
  line L43 (3.883, -0.25) -> (3.883, 0.95)
  line L44 (3.883, 0.95) -> (3.717, 0.95)
  line L45 (3.717, 0.95) -> (3.717, -0.25)
  line L46 (3.717, -0.25) -> (3.483, -0.25)
  line L47 (3.483, -0.25) -> (3.483, 0.95)
  line L48 (3.483, 0.95) -> (3.317, 0.95)
  line L49 (3.317, 0.95) -> (3.317, -0.25)
  line L50 (3.317, -0.25) -> (3.083, -0.25)
  line L51 (3.083, -0.25) -> (3.083, 0.95)
  line L52 (3.083, 0.95) -> (2.917, 0.95)
  line L53 (2.917, 0.95) -> (2.917, -0.25)
  line L54 (2.917, -0.25) -> (2.683, -0.25)
  line L55 (2.683, -0.25) -> (2.683, 0.95)
  line L56 (2.683, 0.95) -> (2.517, 0.95)
  line L57 (2.517, 0.95) -> (2.517, -0.25)
  line L58 (2.517, -0.25) -> (2.283, -0.25)
  line L59 (2.283, -0.25) -> (2.283, 0.95)
  line L60 (2.283, 0.95) -> (2.117, 0.95)
  line L61 (2.117, 0.95) -> (2.117, -0.25)
  line L62 (2.117, -0.25) -> (1.883, -0.25)
  line L63 (1.883, -0.25) -> (1.883, 0.95)
  line L64 (1.883, 0.95) -> (1.717, 0.95)
  line L65 (1.717, 0.95) -> (1.717, -0.25)
  line L66 (1.717, -0.25) -> (1.483, -0.25)
  line L67 (1.483, -0.25) -> (1.483, 0.95)
  line L68 (1.483, 0.95) -> (1.317, 0.95)
  line L69 (1.317, 0.95) -> (1.317, -0.25)
  line L70 (1.317, -0.25) -> (1.083, -0.25)
  line L71 (1.083, -0.25) -> (1.083, 0.95)
  line L72 (1.083, 0.95) -> (0.917, 0.95)
  line L73 (0.917, 0.95) -> (0.917, -0.25)
  line L74 (0.917, -0.25) -> (0.683, -0.25)
  line L75 (0.683, -0.25) -> (0.683, 0.95)
  line L76 (0.683, 0.95) -> (0.517, 0.95)
  line L77 (0.517, 0.95) -> (0.517, -0.25)
  line L78 (0.517, -0.25) -> (0.283, -0.25)
  line L79 (0.283, -0.25) -> (0.283, 0.95)
  line L80 (0.283, 0.95) -> (0.117, 0.95)
  line L81 (0.117, 0.95) -> (0.117, -0.25)
  line L82 (0.117, -0.25) -> (-0.117, -0.25)
  line L83 (-0.117, -0.25) -> (-0.117, 0.95)
  line L84 (-0.117, 0.95) -> (-0.283, 0.95)
  line L85 (-0.283, 0.95) -> (-0.283, -0.25)
  line L86 (-0.283, -0.25) -> (-0.517, -0.25)
  line L87 (-0.517, -0.25) -> (-0.517, 0.95)
  line L88 (-0.517, 0.95) -> (-0.683, 0.95)
  line L89 (-0.683, 0.95) -> (-0.683, -0.25)
  line L90 (-0.683, -0.25) -> (-0.917, -0.25)
  line L91 (-0.917, -0.25) -> (-0.917, 0.95)
  line L92 (-0.917, 0.95) -> (-1.083, 0.95)
  line L93 (-1.083, 0.95) -> (-1.083, -0.25)
  line L94 (-1.083, -0.25) -> (-1.317, -0.25)
  line L95 (-1.317, -0.25) -> (-1.317, 0.95)
  line L96 (-1.317, 0.95) -> (-1.483, 0.95)
  line L97 (-1.483, 0.95) -> (-1.483, -0.25)
  line L98 (-1.483, -0.25) -> (-1.717, -0.25)
  line L99 (-1.717, -0.25) -> (-1.717, 0.95)
  line L100 (-1.717, 0.95) -> (-1.883, 0.95)
  line L101 (-1.883, 0.95) -> (-1.883, -0.25)
  line L102 (-1.883, -0.25) -> (-2.117, -0.25)
  line L103 (-2.117, -0.25) -> (-2.117, 0.95)
  line L104 (-2.117, 0.95) -> (-2.283, 0.95)
  line L105 (-2.283, 0.95) -> (-2.283, -0.25)
  line L106 (-2.283, -0.25) -> (-2.517, -0.25)
  line L107 (-2.517, -0.25) -> (-2.517, 0.95)
  line L108 (-2.517, 0.95) -> (-2.683, 0.95)
  line L109 (-2.683, 0.95) -> (-2.683, -0.25)
  line L110 (-2.683, -0.25) -> (-2.917, -0.25)
  line L111 (-2.917, -0.25) -> (-2.917, 0.95)
  line L112 (-2.917, 0.95) -> (-3.083, 0.95)
  line L113 (-3.083, 0.95) -> (-3.083, -0.25)
  line L114 (-3.083, -0.25) -> (-3.317, -0.25)
  line L115 (-3.317, -0.25) -> (-3.317, 0.95)
  line L116 (-3.317, 0.95) -> (-3.483, 0.95)
  line L117 (-3.483, 0.95) -> (-3.483, -0.25)
  line L118 (-3.483, -0.25) -> (-3.717, -0.25)
  line L119 (-3.717, -0.25) -> (-3.717, 0.95)
  line L120 (-3.717, 0.95) -> (-3.883, 0.95)
  line L121 (-3.883, 0.95) -> (-3.883, -0.25)
  line L122 (-3.883, -0.25) -> (-4.117, -0.25)
  line L123 (-4.117, -0.25) -> (-4.117, 0.95)
  line L124 (-4.117, 0.95) -> (-4.283, 0.95)
  line L125 (-4.283, 0.95) -> (-4.283, -0.25)
  line L126 (-4.283, -0.25) -> (-4.517, -0.25)
  line L127 (-4.517, -0.25) -> (-4.517, 0.95)
  line L128 (-4.517, 0.95) -> (-4.683, 0.95)
  line L129 (-4.683, 0.95) -> (-4.683, -0.25)
  line L130 (-4.683, -0.25) -> (-4.917, -0.25)
  line L131 (-4.917, -0.25) -> (-4.917, 0.95)
  line L132 (-4.917, 0.95) -> (-5.083, 0.95)
  line L133 (-5.083, 0.95) -> (-5.083, -0.25)
  line L134 (-5.083, -0.25) -> (-5.317, -0.25)
  line L135 (-5.317, -0.25) -> (-5.317, 0.95)
  line L136 (-5.317, 0.95) -> (-5.483, 0.95)
  line L137 (-5.483, 0.95) -> (-5.483, -0.25)
  line L138 (-5.483, -0.25) -> (-5.717, -0.25)
  line L139 (-5.717, -0.25) -> (-5.717, 0.95)
  line L140 (-5.717, 0.95) -> (-5.883, 0.95)
  line L141 (-5.883, 0.95) -> (-5.883, -0.25)
  line L142 (-5.883, -0.25) -> (-6.117, -0.25)
  line L143 (-6.117, -0.25) -> (-6.117, 0.95)
  line L144 (-6.117, 0.95) -> (-6.283, 0.95)
  line L145 (-6.283, 0.95) -> (-6.283, -0.25)
  line L146 (-6.283, -0.25) -> (-6.517, -0.25)
  line L147 (-6.517, -0.25) -> (-6.517, 0.95)
  line L148 (-6.517, 0.95) -> (-6.683, 0.95)
  line L149 (-6.683, 0.95) -> (-6.683, -0.25)
  line L150 (-6.683, -0.25) -> (-6.917, -0.25)
  line L151 (-6.917, -0.25) -> (-6.917, 0.95)
  line L152 (-6.917, 0.95) -> (-7.083, 0.95)
  line L153 (-7.083, 0.95) -> (-7.083, -0.25)
  line L154 (-7.083, -0.25) -> (-7.317, -0.25)
  line L155 (-7.317, -0.25) -> (-7.317, 0.95)
  line L156 (-7.317, 0.95) -> (-7.483, 0.95)
  line L157 (-7.483, 0.95) -> (-7.483, -0.25)
  line L158 (-7.483, -0.25) -> (-7.717, -0.25)
  line L159 (-7.717, -0.25) -> (-7.717, 0.95)
  line L160 (-7.717, 0.95) -> (-7.883, 0.95)
  line L161 (-7.883, 0.95) -> (-7.883, -1)
  constraints: 324 end point
extrude "Extrusion11" cut sketch "Sketch_19" along normal blind 1.7
sketch "Sketch_20" plane through (0, 0, 0) normal (1, 0, 0) x (0, 1, 0)
  line L0 (0.9, 2.175) -> (1.3717, 2)
  arc A0 (1.3717, 2) -> (1.65, 1.95) centre (1.65, 2.75) ccw
  line L1 (1.65, 1.95) -> (3.75, 1.95)
  line L2 (3.75, 1.95) -> (3.75, -1.95)
  line L3 (3.75, -1.95) -> (1.65, -1.95)
  arc A1 (1.65, -1.95) -> (1.3717, -2) centre (1.65, -2.75) ccw
  line L4 (1.3717, -2) -> (0.9, -2.175)
  line L5 (0.9, -2.175) -> (4.4, -2.175)
  line L6 (4.4, -2.175) -> (4.4, 2.175)
  line L7 (4.4, 2.175) -> (0.9, 2.175)
  constraints: 16 end point, 4 point on circle, 2 centre point
extrude "Extrusion12" cut sketch "Sketch_20" along normal mid plane 23.54
sketch "Sketch_21" plane through (0, 0, 0) normal (1, 0, 0) x (0, 1, 0)
  line L0 (0.45, 2.175) -> (-1, 2.175)
  line L1 (-1, 2.175) -> (-1, -2.175)
  line L2 (-1, -2.175) -> (0.45, -2.175)
  line L3 (0.45, -2.175) -> (0.35, -2.1173)
  line L4 (0.35, -2.1173) -> (0.35, -1.775)
  line L5 (0.35, -1.775) -> (0, -1.775)
  line L6 (0, -1.775) -> (0, 1.775)
  line L7 (0, 1.775) -> (0.35, 1.775)
  line L8 (0.35, 1.775) -> (0.35, 2.1173)
  line L9 (0.35, 2.1173) -> (0.45, 2.175)
  constraints: 20 end point
extrude "Extrusion13" cut sketch "Sketch_21" along normal mid plane 23.54
sketch "Sketch_22" plane through (0, 0, 0) normal (0, 1, 0) x (1, 0, 0)
  line L0 (-10.06, 2.175) -> (-10.06, -2.175)
  line L1 (-10.06, -2.175) -> (-8.63, -2.175)
  line L2 (-8.63, -2.175) -> (-8.63, -1.405)
  arc A0 (-8.63, -1.405) -> (-8.83, -1.205) centre (-8.83, -1.405) ccw
  line L3 (-8.83, -1.205) -> (-9.56, -1.205)
  line L4 (-9.56, -1.205) -> (-9.56, 1.205)
  line L5 (-9.56, 1.205) -> (-8.83, 1.205)
  arc A1 (-8.83, 1.205) -> (-8.63, 1.405) centre (-8.83, 1.405) ccw
  line L6 (-8.63, 1.405) -> (-8.63, 2.175)
  line L7 (-8.63, 2.175) -> (-10.06, 2.175)
  constraints: 16 end point, 4 point on circle, 2 centre point
extrude "Extrusion14" cut sketch "Sketch_22" along normal blind 0.45
sketch "Sketch_23" plane through (-8.23, 0, 0) normal (1, 0, 0) x (0, 0, -1)
  line L0 (-2.175, 4.4) -> (-2.175, 0.9)
  line L1 (-2.175, 0.9) -> (-2, 0.9)
  arc A0 (-2, 0.9) -> (-1.9, 1) centre (-2, 1) ccw
  line L2 (-1.9, 1) -> (-1.9, 1.39)
  arc A1 (-1.54, 1.75) -> (-1.9, 1.39) centre (-1.54, 1.39) ccw
  line L3 (-1.54, 1.75) -> (-1.54, 3.75)
  line L4 (-1.54, 3.75) -> (1.54, 3.75)
  line L5 (1.54, 3.75) -> (1.54, 1.75)
  arc A2 (1.9, 1.39) -> (1.54, 1.75) centre (1.54, 1.39) ccw
  line L6 (1.9, 1.39) -> (1.9, 1)
  arc A3 (1.9, 1) -> (2, 0.9) centre (2, 1) ccw
  line L7 (2, 0.9) -> (2.175, 0.9)
  line L8 (2.175, 0.9) -> (2.175, 4.4)
  line L9 (2.175, 4.4) -> (-2.175, 4.4)
  constraints: 20 end point, 8 point on circle, 4 centre point
extrude "Extrusion15" cut sketch "Sketch_23" against normal blind 0.5
sketch "Sketch_24" plane through (8.23, 0, 0) normal (1, 0, 0) x (0, 0, -1)
  line L0 (-2.175, 4.25) -> (-2.175, 0.75)
  line L1 (-2.175, 0.75) -> (-2, 0.75)
  arc A0 (-2, 0.75) -> (-1.9, 0.85) centre (-2, 0.85) ccw
  line L2 (-1.9, 0.85) -> (-1.9, 1.39)
  arc A1 (-1.54, 1.75) -> (-1.9, 1.39) centre (-1.54, 1.39) ccw
  line L3 (-1.54, 1.75) -> (-1.54, 3.75)
  line L4 (-1.54, 3.75) -> (1.54, 3.75)
  line L5 (1.54, 3.75) -> (1.54, 1.75)
  arc A2 (1.9, 1.39) -> (1.54, 1.75) centre (1.54, 1.39) ccw
  line L6 (1.9, 1.39) -> (1.9, 0.85)
  arc A3 (1.9, 0.85) -> (2, 0.75) centre (2, 0.85) ccw
  line L7 (2, 0.75) -> (2.175, 0.75)
  line L8 (2.175, 0.75) -> (2.175, 4.25)
  line L9 (2.175, 4.25) -> (-2.175, 4.25)
  constraints: 20 end point, 8 point on circle, 4 centre point
extrude "Extrusion16" cut sketch "Sketch_24" along normal blind 0.5
sketch "Sketch_25" plane through (0, 2.725, 0) normal (0, 1, 0) x (1, 0, 0)
  line L0 (-6.5, -1.54) -> (-6.5, -2.175)
  line L1 (-6.5, -2.175) -> (-5.5, -2.175)
  line L2 (-5.5, -2.175) -> (-5.5, -1.54)
  line L3 (-5.5, -1.54) -> (-6.5, -1.54)
  constraints: 8 end point
extrude "Extrusion17" cut sketch "Sketch_25" against normal blind 0.6
sketch "Sketch_26" plane through (0, 2.725, 0) normal (0, 1, 0) x (1, 0, 0)
  line L0 (-6.5, 1.54) -> (-5.5, 1.54)
  line L1 (-5.5, 1.54) -> (-5.5, 2.175)
  line L2 (-5.5, 2.175) -> (-6.5, 2.175)
  line L3 (-6.5, 2.175) -> (-6.5, 1.54)
  constraints: 8 end point
extrude "Extrusion18" cut sketch "Sketch_26" against normal blind 0.6
sketch "Sketch_27" plane through (0, 2.725, 0) normal (0, 1, 0) x (1, 0, 0)
  line L0 (-6.5, -3.175) -> (7.5, -3.175)
  line L1 (7.5, -3.175) -> (7.5, -2.175)
  line L2 (7.5, -2.175) -> (6.5, -2.175)
  line L3 (6.5, -2.175) -> (6.5, -1.54)
  line L4 (6.5, -1.54) -> (5.5, -1.54)
  line L5 (5.5, -1.54) -> (5.5, -2.175)
  line L6 (5.5, -2.175) -> (4.5, -2.175)
  line L7 (4.5, -2.175) -> (4.5, -1.54)
  line L8 (4.5, -1.54) -> (3.5, -1.54)
  line L9 (3.5, -1.54) -> (3.5, -2.175)
  line L10 (3.5, -2.175) -> (2.5, -2.175)
  line L11 (2.5, -2.175) -> (2.5, -1.54)
  line L12 (2.5, -1.54) -> (1.5, -1.54)
  line L13 (1.5, -1.54) -> (1.5, -2.175)
  line L14 (1.5, -2.175) -> (0.5, -2.175)
  line L15 (0.5, -2.175) -> (0.5, -1.54)
  line L16 (0.5, -1.54) -> (-0.5, -1.54)
  line L17 (-0.5, -1.54) -> (-0.5, -2.175)
  line L18 (-0.5, -2.175) -> (-1.5, -2.175)
  line L19 (-1.5, -2.175) -> (-1.5, -1.54)
  line L20 (-1.5, -1.54) -> (-2.5, -1.54)
  line L21 (-2.5, -1.54) -> (-2.5, -2.175)
  line L22 (-2.5, -2.175) -> (-3.5, -2.175)
  line L23 (-3.5, -2.175) -> (-3.5, -1.54)
  line L24 (-3.5, -1.54) -> (-4.5, -1.54)
  line L25 (-4.5, -1.54) -> (-4.5, -2.175)
  line L26 (-4.5, -2.175) -> (-5.5, -2.175)
  line L27 (-5.5, -2.175) -> (-5.5, -1.54)
  line L28 (-5.5, -1.54) -> (-6.5, -1.54)
  line L29 (-6.5, -1.54) -> (-6.5, -3.175)
  constraints: 60 end point
extrude "Extrusion19" cut sketch "Sketch_27" against normal blind 0.6
sketch "Sketch_28" plane through (0, 2.725, 0) normal (0, 1, 0) x (1, 0, 0)
  line L0 (-6.5, 3.175) -> (-6.5, 1.54)
  line L1 (-6.5, 1.54) -> (-5.5, 1.54)
  line L2 (-5.5, 1.54) -> (-5.5, 2.175)
  line L3 (-5.5, 2.175) -> (-4.5, 2.175)
  line L4 (-4.5, 2.175) -> (-4.5, 1.54)
  line L5 (-4.5, 1.54) -> (-3.5, 1.54)
  line L6 (-3.5, 1.54) -> (-3.5, 2.175)
  line L7 (-3.5, 2.175) -> (-2.5, 2.175)
  line L8 (-2.5, 2.175) -> (-2.5, 1.54)
  line L9 (-2.5, 1.54) -> (-1.5, 1.54)
  line L10 (-1.5, 1.54) -> (-1.5, 2.175)
  line L11 (-1.5, 2.175) -> (-0.5, 2.175)
  line L12 (-0.5, 2.175) -> (-0.5, 1.54)
  line L13 (-0.5, 1.54) -> (0.5, 1.54)
  line L14 (0.5, 1.54) -> (0.5, 2.175)
  line L15 (0.5, 2.175) -> (1.5, 2.175)
  line L16 (1.5, 2.175) -> (1.5, 1.54)
  line L17 (1.5, 1.54) -> (2.5, 1.54)
  line L18 (2.5, 1.54) -> (2.5, 2.175)
  line L19 (2.5, 2.175) -> (3.5, 2.175)
  line L20 (3.5, 2.175) -> (3.5, 1.54)
  line L21 (3.5, 1.54) -> (4.5, 1.54)
  line L22 (4.5, 1.54) -> (4.5, 2.175)
  line L23 (4.5, 2.175) -> (5.5, 2.175)
  line L24 (5.5, 2.175) -> (5.5, 1.54)
  line L25 (5.5, 1.54) -> (6.5, 1.54)
  line L26 (6.5, 1.54) -> (6.5, 2.175)
  line L27 (6.5, 2.175) -> (7.5, 2.175)
  line L28 (7.5, 2.175) -> (7.5, 3.175)
  line L29 (7.5, 3.175) -> (-6.5, 3.175)
  constraints: 60 end point
extrude "Extrusion20" cut sketch "Sketch_28" against normal blind 0.6
sketch "Sketch_29" plane through (8.58, 0, 0) normal (1, 0, 0) x (0, 0, -1)
  line L0 (1.04, 0.2) -> (1.96, 0.2)
  line L1 (1.96, 0.2) -> (1.5, 1)
  line L2 (1.5, 1) -> (1.04, 0.2)
  constraints: 6 end point
extrude "Extrusion21" cut sketch "Sketch_29" along normal mid plane 0.1
ref_plane "socket_to_dummy_XY" through (0, 0, 0) normal (0, -1, 0) x (1, 0, 0)
ref_plane "socket_to_dummy_YZ" through (0, 0, 0) normal (1, 0, 0) x (0, 0, 1)
ref_plane "socket_to_dummy_ZX" through (0, 0, 0) normal (0, 0, 1) x (0, -1, 0)
ref_plane "socket_to_pad_XY" through (0, 2.725, 0) normal (0, 1, 0) x (1, 0, 0)
ref_plane "socket_to_pad_YZ" through (0, 2.725, 0) normal (1, 0, 0) x (0, 0, -1)
ref_plane "socket_to_pad_ZX" through (0, 2.725, 0) normal (0, 0, -1) x (0, 1, 0)
body "Solid1"
